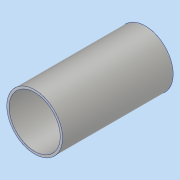
# Autodesk Inventor part: pistonTank
Saved by Autodesk Inventor 2017.3 (Build 213256000, 256)
## iProperties
Created: 2016-11-20
Part Number: pistonTank
Material: Aluminum 6061
Document SubType Name: Modeling
Designer: techn
Density: 2.7 g/cm^3
Appearance: Aluminum - Flat
Mass: 207.673 g
Surface Area: 792.921 cm^2
Volume: 220.929 cm^3
Author: techn
Autodesk Inventor part; units mm, degrees
ref_plane "YZ Plane" through (0, 0, 0) normal (1, 0, 0) x (0, 1, 0)
ref_plane "XZ Plane" through (0, 0, 0) normal (0, 1, 0) x (-1, 0, 0)
ref_plane "XY Plane" through (0, 0, 0) normal (0, 0, 1) x (1, 0, 0)
sketch "Sketch1" plane through (0, 0, 0) normal (0, 0, 1) x (1, 0, 0)
  circle A0 centre (0, 0) radius 38.1
  circle A1 centre (0, 0) radius 34.925
  dimension "d0" = 76.2
  dimension "d1" = 69.85
  constraints: 2 centre point, 2 coincident
  measures "d0" diameter of A0
  measures "d1" diameter of A1
extrude "Extrusion1" add sketch "Sketch1" along normal blind 151.13
body "Solid1"
